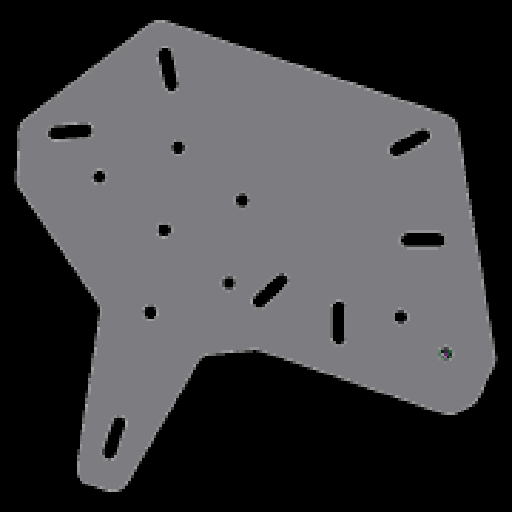
# Autodesk Inventor part: UpperLeg2
Saved by Autodesk Inventor 2025.2 (Build 292293000, 293)
## iProperties
Created: 2020-05-16
Part Number: UpperLeg2
Material: Generic
Document SubType Name: Sheet Metal
Designer: valer
Density: 1 g/cm^3
Sheet Metal Rule: Default
Appearance: Default
Author: valer
Autodesk Inventor part; units mm, degrees
ref_plane "YZ Plane" through (0, 0, 0) normal (1, 0, 0) x (0, 1, 0)
ref_plane "XZ Plane" through (0, 0, 0) normal (0, 1, 0) x (-1, 0, 0)
ref_plane "XY Plane" through (0, 0, 0) normal (0, 0, 1) x (1, 0, 0)
sketch "Base" plane through (0, 0, 0) normal (0, 0, 1) x (1, 0, 0)
  circle A0 centre (6.3437, -0.0043) radius 44.7044
  line L0 (-53.391, 43.8831) -> (3.4518, 87.3031)
  line L1 (3.4518, 87.3031) -> (126.7242, 46.1195)
  line L2 (21.9665, -51.542) -> (-11.8651, -109.4379)
  line L3 (134.9457, -71.4872) -> (143.2137, -54.1334)
  line L4 (44.7126, -49.2622) -> (124.7112, -76.8356)
  line L5 (44.7126, -49.2622) -> (21.9665, -51.542)
  line L6 (126.7242, 46.1195) -> (143.2137, -54.1334)
  line L7 (134.9457, -71.4872) -> (124.7112, -76.8356)
  line L8 (-30.3614, -103.0627) -> (-11.8651, -109.4379)
  line L9 (-30.3614, -103.0627) -> (-19.8027, -31.8971)
  line L10 (-54.6035, 18.8674) -> (-53.391, 43.8831)
  line L11 (-54.6035, 18.8674) -> (-19.8027, -31.8971)
  line L12 (-94.1669, 0) -> (182.7771, 0) construction
  circle A1 centre (6.3437, -0.0043) radius 3
  circle A2 centre (103.8642, -35.9814) radius 3
  line L13 (126.7242, 46.1195) -> (-19.8027, -31.8971) construction
  line L14 (3.4518, 87.3031) -> (33.3396, -50.4021) construction
  line L15 (-53.9972, 31.3753) -> (126.7242, 46.1195) construction
  line L16 (134.969, -4.007) -> (-37.2031, -6.5149) construction
  line L17 (-21.1132, -106.2503) -> (39.5241, 75.2519) construction
  line L18 (78.4642, -60.8955) -> (78.4642, 62.2425) construction
  line L19 (21.9665, -51.542) -> (126.7242, 46.1195) construction
  line L20 (0, 0) -> (-53.391, 43.8831) construction
  circle A3 centre (-20.3518, 21.9373) radius 3
  circle A4 centre (6.3437, -0.0043) radius 34.5555 construction
  circle A5 centre (-26.006, -12.1525) radius 3
  circle A6 centre (0.6895, -34.0941) radius 3
  circle A7 centre (33.0392, -21.9459) radius 3
  circle A8 centre (38.6934, 12.1439) radius 3
  circle A9 centre (11.9979, 34.0855) radius 3
  line L21 (113.2722, 38.9571) -> (102.0622, 32.9885) construction
  line L22 (111.8623, 41.6052) -> (100.6522, 35.6365)
  line L23 (103.4721, 30.3404) -> (114.6821, 36.3091)
  arc A10 (114.6821, 36.3091) -> (111.8623, 41.6052) centre (113.2722, 38.9571) ccw
  arc A11 (100.6522, 35.6365) -> (103.4721, 30.3404) centre (102.0622, 32.9885) ccw
  line L24 (119.5611, -4.2314) -> (106.8611, -4.2314) construction
  line L25 (119.5611, -1.2314) -> (106.8611, -1.2314)
  line L26 (106.8611, -7.2314) -> (119.5611, -7.2314)
  arc A12 (119.5611, -7.2314) -> (119.5611, -1.2314) centre (119.5611, -4.2314) ccw
  arc A13 (106.8611, -1.2314) -> (106.8611, -7.2314) centre (106.8611, -4.2314) ccw
  line L27 (6.6843, 72.4098) -> (9.378, 59.9988) construction
  line L28 (3.7525, 71.7735) -> (6.4462, 59.3625)
  line L29 (12.3097, 60.6351) -> (9.616, 73.0462)
  arc A14 (9.616, 73.0462) -> (3.7525, 71.7735) centre (6.6843, 72.4098) ccw
  arc A15 (6.4462, 59.3625) -> (12.3097, 60.6351) centre (9.378, 59.9988) ccw
  line L30 (-16.2839, -91.795) -> (-12.2597, -79.7494) construction
  line L31 (-13.4385, -92.7456) -> (-9.4142, -80.7)
  line L32 (-15.1051, -78.7988) -> (-19.1293, -90.8444)
  arc A16 (-19.1293, -90.8444) -> (-13.4385, -92.7456) centre (-16.2839, -91.795) ccw
  arc A17 (-9.4142, -80.7) -> (-15.1051, -78.7988) centre (-12.2597, -79.7494) ccw
  line L33 (78.4642, -44.7756) -> (78.4642, -32.0756) construction
  line L34 (75.4642, -44.7756) -> (75.4642, -32.0756)
  line L35 (81.4642, -32.0756) -> (81.4642, -44.7756)
  arc A18 (75.4642, -44.7756) -> (81.4642, -44.7756) centre (78.4642, -44.7756) ccw
  arc A19 (81.4642, -32.0756) -> (75.4642, -32.0756) centre (78.4642, -32.0756) ccw
  line L36 (-38.6678, 39.9478) -> (-26.0099, 40.9805) construction
  line L37 (-38.4239, 36.9578) -> (-25.766, 37.9905)
  line L38 (-26.2538, 43.9706) -> (-38.9118, 42.9379)
  arc A20 (-38.9118, 42.9379) -> (-38.4239, 36.9578) centre (-38.6678, 39.9478) ccw
  arc A21 (-25.766, 37.9905) -> (-26.2538, 43.9706) centre (-26.0099, 40.9805) ccw
  line L39 (45.5702, -29.5373) -> (54.8596, -20.8771) construction
  line L40 (47.6159, -31.7316) -> (56.9053, -23.0715)
  line L41 (52.8139, -18.6828) -> (43.5245, -27.3429)
  arc A22 (43.5245, -27.3429) -> (47.6159, -31.7316) centre (45.5702, -29.5373) ccw
  arc A23 (56.9053, -23.0715) -> (52.8139, -18.6828) centre (54.8596, -20.8771) ccw
  line L42 (-38.6678, 39.9478) -> (-53.391, 43.8831) construction
  circle A24 centre (122.4612, -51.192) radius 3
  point P0 (107.6672, 35.9728)
  point P1 (113.2111, -4.2314)
  point P2 (8.0311, 66.2043)
  point P3 (-14.2718, -85.7722)
  point P4 (78.4642, -38.4256)
  point P5 (-32.3389, 40.4642)
  point P6 (50.2149, -25.2072)
  dimension "d48" = 69.111
  dimension "d1" = 89.4088
  dimension "d2" = 55.568
  dimension "d3" = 37.094
  dimension "d4" = 120.3
  dimension "d5" = 81.561
  dimension "d6" = 160.982
  dimension "d7" = 133.392
  dimension "d8" = 143.066
  dimension "d9" = 145.185
  dimension "d10" = 124.151
  dimension "d11" = 130.15
  dimension "d12" = 142.793
  dimension "d13" = 117.814
  dimension "d14" = 19.5642
  dimension "d15" = 25.0158
  dimension "d16" = 71.529
  dimension "d17" = 61.5478
  dimension "d18" = 129.9699
  dimension "d19" = 101.6
  dimension "d20" = 19.2227
  dimension "d21" = 11.5477
  dimension "d22" = 84.6172
  dimension "d23" = 67.056
  dimension "d24" = 22.86
  dimension "d25" = 39.5986
  dimension "d26" = 71.1371
  dimension "d29" = 6
  dimension "d30" = 6
  dimension "d31" = 48.26
  dimension "d32" = 6
  dimension "d35" = 360
  dimension "d37" = 6
  dimension "d38" = 6
  dimension "d39" = 15.24
  dimension "d40" = 12.7
  dimension "d41" = 15.24
  dimension "d43" = 15.24
  dimension "d44" = 15.24
  dimension "d45" = 15.24
  dimension "d46" = 15.7016
  dimension "d49" = 140.583
  dimension "d50" = 4.2314
  dimension "d51" = 91.5631
  dimension "d52" = 12.1439
  dimension "d53" = 0
  dimension "d60" = 126.024
  dimension "d61" = 155.259
  dimension "d63" = 15.24
  dimension "d64" = 12.0647
  dimension "d67" = 25.4
  dimension "d68" = 31.75
  dimension "d69" = 6
  dimension "d70" = 20
  dimension "d71" = 20
  dimension "d72" = 3
  dimension "d73" = 3
  dimension "d74" = 3
  dimension "d75" = 3
  dimension "d76" = 3
  dimension "d77" = 3
  dimension "d78" = 3
  dimension "d79" = 3
  dimension "d80" = 3
  dimension "d81" = 3
  measures "d1" diameter of A0
  measures "d2" angle of L11 L12
  measures "d3" angle of L1 L11
  measures "d4" angle of L2 L12
  measures "d5" angle of L12 L9
  measures "d6" angle of L12 L4
  measures "d7" angle of L7 L4
  measures "d8" angle of L3 L7
  measures "d9" angle of L6 L3
  measures "d10" angle of L1 L0
  measures "d11" angle of L0 L10
  measures "d12" angle of L11 L10
  measures "d13" angle of L6 L1
  measures "d14" distance of L8.start L2.end
  measures "d15" vertical distance of L10.start L0.start
  measures "d16" distance of L0.start L0.end
  measures "d17" distance of L10.start L9.end
  measures "d18" distance of L0.end L1.end
  measures "d19" distance of L1.end L3.end
  measures "d20" distance of L3.start L3.end
  measures "d21" distance of L3.start L4.end
  measures "d22" distance of L4.start L4.end
  measures "d23" distance of L2.start L2.end
  measures "d24" distance of L4.start L2.start
  measures "d25" distance from line of L11 A0.centre
  measures "d26" distance from line of L0 A0.centre
  measures "d29" diameter of A1
  measures "d30" diameter of A2
  measures "d31" distance from line of L1.end L18
  measures "d32" diameter of A3
  measures "d37" diameter of A11
  measures "d38" diameter of A13
  measures "d39" distance of L1.end L21.start
  measures "d40" distance of L21.start L21.end
  measures "d41" distance from line of L6 L24.start
  measures "d43" distance of L0.end L27.start
  measures "d44" distance from line of L8 L30.start
  measures "d45" distance from line of L4 L33.start
  measures "d46" distance from line of L16 L39.end
  measures "d49" angle of L20 L12
  measures "d50" distance between parallel lines of L24 L12
  measures "d51" distance from line of L12.end L4
  measures "d52" distance from line of A8.centre L12
  measures "d53" distance from line of L20.start L12
  measures "d60" angle of L2 L5
  measures "d61" angle of L4 L5
  measures "d63" distance of L36.start L0.start
  measures "d64" distance from line of L0 L36.start
  measures "d67" distance from line of L18 A2.centre
  measures "d68" vertical distance of A2.centre L24.end
  measures "d69" diameter of A24
  measures "d70" distance from line of L6 A24.centre
  measures "d71" distance from line of L3 A24.centre
  measures "d72" radius of A15
  measures "d73" radius of A14
  measures "d74" radius of A21
  measures "d75" radius of A20
  measures "d76" radius of A22
  measures "d77" radius of A23
  measures "d78" radius of A10
  measures "d79" radius of A19
  measures "d80" radius of A18
  measures "d81" radius of A17
extrude "Plate1" add sketch "Base" along normal blind 5 contours A0 L9 L11 | A0 L11 L10 L0 L1 L6 L3 L7 L4 L5 L2 L8 L9 | A5 picked at (-13.3863, 3.3874)
fillet "OutsideFilletsFeature" radius 6.35 12 edges at (126.7242, 46.1195, 2.5) (3.4518, 87.3031, 2.5) (143.2137, -54.1334, 2.5) (134.9457, -71.4872, 2.5) (124.7112, -76.8356, 2.5) (-11.8651, -109.4379, 2.5) (44.7126, -49.2622, 2.5) (21.9665, -51.542, 2.5) (-30.3614, -103.0627, 2.5) (-19.8027, -31.8971, 2.5) (-54.6035, 18.8674, 2.5) (-53.391, 43.8831, 2.5)
sketch "HandleAttachment" plane through (0, 0, 0) normal (0, 0, -1) x (-1, 0, 0)
  circle A0 centre (-122.4612, -51.192) radius 3 projected
  point P0 (0, 0)
  constraints: 1 coincident
equation "\"d41\" = d39"
equation "\"d43\" = d39"
equation "\"d44\" = d43"
equation "\"d45\" = d43"
equation "\"d47\" = Thickness"
equation "\"Thickness\" = 5"
body "Solid1"
